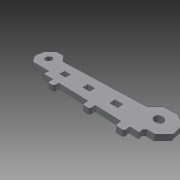
# Autodesk Inventor part: rope_mount_a
Saved by Autodesk Inventor 2014 (Build 180170000, 170)
## iProperties
Created: 2013-12-16
Part Number: rope_mount_a
Material: Generic
Document SubType Name: Modeling
Designer: buben
Density: 1 g/cm^3
Appearance: Anodized - Dark Gray
Author: buben
Autodesk Inventor part; units mm, degrees
ref_plane "YZ Plane" through (0, 0, 0) normal (1, 0, 0) x (0, 1, 0)
ref_plane "XZ Plane" through (0, 0, 0) normal (0, 1, 0) x (-1, 0, 0)
ref_plane "XY Plane" through (0, 0, 0) normal (0, 0, 1) x (1, 0, 0)
sketch "Sketch1" plane through (0, 0, 0) normal (0, 0, 1) x (1, 0, 0)
  circle A0 centre (-18.4853, 20.4853) radius 4.25
  circle A1 centre (107.6147, 20.4853) radius 4.25
  line L0 (-33.4853, 26.4853) -> (-33.4853, 14.4853)
  line L1 (-33.4853, 26.4853) -> (-25, 34.9706)
  line L2 (-33.4853, 14.4853) -> (-25, 6)
  line L3 (-25, 34.9706) -> (114.1294, 34.9706)
  line L4 (114.1294, 34.9706) -> (122.6147, 26.4853)
  line L5 (122.6147, 26.4853) -> (122.6147, 14.4853)
  line L6 (122.6147, 14.4853) -> (114.1294, 6)
  circle A2 centre (-18.4853, 20.4853) radius 13 construction
  circle A3 centre (-18.4853, 20.4853) radius 17 construction
  line L7 (-25, 6) -> (0, 6)
  line L8 (0, 6) -> (0, 0)
  line L9 (114.1294, 6) -> (105.6147, 6)
  line L10 (105.6147, 6) -> (105.6147, 0)
  line L11 (105.6147, 0) -> (0, 0)
  point P0 (0, 0)
  point P1 (-33.4853, 20.4853)
  dimension "d0" = 8.5
  dimension "d1" = 126.1
  dimension "d2" = 45
  dimension "d3" = 12
  dimension "d4" = 26
  dimension "d5" = 34
  dimension "d6" = 15
  dimension "d7" = 6
  dimension "d10" = 15
  dimension "d18" = 2
  dimension "d19" = 25
  constraints: 24 end point, 8 perpendicular, 4 centre point, 4 horizontal alignment, 3 coincident, 3 equal length, 2 parallel, 1 equal radius, 1 midpoint, 1 vertical
  measures "d0" diameter of A0
  measures "d1" distance of A1.centre A0.centre
  measures "d2" angle of L0 L1
  measures "d3" distance of L0.start L0.end
  measures "d4" diameter of A2
  measures "d5" diameter of A3
  measures "d6" distance from line of A0.centre L0
  measures "d7" distance of L7.end L8.end
  measures "d10" distance from line of L5 A1.centre
  measures "d18" distance from line of L10 A1.centre
  measures "d19" distance of L2.end L7.end
extrude "Extrusion1" add sketch "Sketch1" along normal blind 6
sketch "Sketch2" plane through (0, 0, 6) normal (0, 0, 1) x (1, 0, 0)
  line L0 (114.1294, 34.9706) -> (-25, 34.9706) projected
  line L1 (-25, 34.9706) -> (-33.4853, 26.4853) projected
  line L2 (-13, 34.9706) -> (-4.5147, 26.4853)
  line L3 (-4.5147, 26.4853) -> (93.6442, 26.4853)
  line L4 (93.6442, 26.4853) -> (102.1294, 34.9706)
  point P0 (-33.4853, 14.4853)
  dimension "d13" = 12
  dimension "d14" = 12
  dimension "d15" = 12
  constraints: 6 end point, 2 perpendicular, 2 point on line, 1 horizontal alignment, 1 parallel
  measures "d13" distance of L1.end point (-33.485, 14.485)
  measures "d14" distance of L2.start L0.end
  measures "d15" distance of L0.start L4.end
extrude "Extrusion2" cut sketch "Sketch2" against normal blind 6
sketch "Sketch3" plane through (0, 0, 6) normal (0, 0, 1) x (1, 0, 0)
  line L0 (0, 0) -> (105.6147, 0) projected
  line L1 (93.6442, 26.4853) -> (-4.5147, 26.4853) projected
  line L2 (40.5647, 16) -> (48.5647, 16)
  line L3 (48.5647, 16) -> (48.5647, 10)
  line L4 (48.5647, 10) -> (40.5647, 10)
  line L5 (40.5647, 10) -> (40.5647, 16)
  line L6 (10.5647, 16) -> (18.5647, 16)
  line L7 (18.5647, 16) -> (18.5647, 10)
  line L8 (18.5647, 10) -> (10.5647, 10)
  line L9 (10.5647, 10) -> (10.5647, 16)
  line L10 (70.5647, 16) -> (78.5647, 16)
  line L11 (78.5647, 16) -> (78.5647, 10)
  line L12 (78.5647, 10) -> (70.5647, 10)
  line L13 (70.5647, 10) -> (70.5647, 16)
  point P0 (44.5647, 16)
  point P1 (44.5647, 26.4853)
  dimension "d20" = 8
  dimension "d21" = 6
  dimension "d22" = 8
  dimension "d23" = 8
  dimension "d24" = 10
  dimension "d25" = 22
  dimension "d26" = 22
  constraints: 24 end point, 6 parallel, 4 collinear, 3 horizontal, 3 perpendicular, 2 midpoint, 1 vertical alignment
  measures "d20" distance of L6.start L6.end
  measures "d21" distance of L8.end L6.start
  measures "d22" distance of L2.start L2.end
  measures "d23" distance of L10.start L10.end
  measures "d24" distance between parallel lines of L0 L8
  measures "d25" distance between parallel lines of L5 L7
  measures "d26" distance between parallel lines of L13 L3
extrude "Extrusion3" cut sketch "Sketch3" against normal through all
sketch "Sketch4" plane through (0, 0, 6) normal (0, 0, 1) x (1, 0, 0)
  line L0 (0, 0) -> (105.6147, 0) projected
  line L1 (97.6147, 0) -> (89.6147, 0)
  line L2 (89.6147, 0) -> (89.6147, -4)
  line L3 (91.6147, -6) -> (95.6147, -6)
  line L4 (97.6147, -4) -> (97.6147, 0)
  line L5 (64.6147, 0) -> (56.6147, 0)
  line L6 (56.6147, 0) -> (56.6147, -4)
  line L7 (58.6147, -6) -> (62.6147, -6)
  line L8 (64.6147, -4) -> (64.6147, 0)
  line L9 (21.6147, 0) -> (13.6147, 0)
  line L10 (13.6147, 0) -> (13.6147, -4)
  line L11 (15.6147, -6) -> (19.6147, -6)
  line L12 (21.6147, -4) -> (21.6147, 0)
  arc A0 (13.6147, -4) -> (15.6147, -6) centre (15.6147, -4) ccw
  arc A1 (19.6147, -6) -> (21.6147, -4) centre (19.6147, -4) ccw
  arc A2 (56.6147, -4) -> (58.6147, -6) centre (58.6147, -4) ccw
  arc A3 (62.6147, -6) -> (64.6147, -4) centre (62.6147, -4) ccw
  arc A4 (89.6147, -4) -> (91.6147, -6) centre (91.6147, -4) ccw
  arc A5 (95.6147, -6) -> (97.6147, -4) centre (95.6147, -4) ccw
  dimension "d29" = 2
  dimension "d30" = 8
  dimension "d31" = 8
  dimension "d32" = 8
  dimension "d33" = 6
  dimension "d34" = 8
  dimension "d35" = 25
  dimension "d36" = 35
  constraints: 24 end point, 12 point on circle, 12 tangent, 6 centre point, 6 parallel, 5 equal radius, 3 horizontal, 3 perpendicular, 3 point on line, 2 collinear
  measures "d29" radius of A0
  measures "d30" distance between parallel lines of L12 L10
  measures "d31" distance between parallel lines of L8 L6
  measures "d32" distance between parallel lines of L4 L2
  measures "d33" distance between parallel lines of L0 L11
  measures "d34" distance from line of L0.end L4
  measures "d35" distance between parallel lines of L2 L8
  measures "d36" distance between parallel lines of L12 L6
extrude "Extrusion4" add sketch "Sketch4" against normal blind 6
chamfer "Chamfer1" distance 2 angle 45 1 edges at (105.6147, 6, 3)
equation "\"d14\" = d13"
equation "\"d15\" = d14"
equation "\"d26\" = d25"
body "Solid1"
